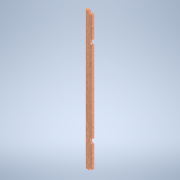
# Autodesk Inventor part: ReedRail
Saved by Autodesk Inventor 2022.2 (Build 262287000, 287)
## iProperties
Created: 2023-02-20
Part Number: ReedRail
Material: Wood (Oak)
Document SubType Name: Modeling
Designer: jaege
Density: 0.76 g/cm^3
Appearance: Red Oak - Natural Low Gloss
Author: jaege
Autodesk Inventor part; units mm, degrees
ref_plane "YZ Plane" through (0, 0, 0) normal (1, 0, 0) x (0, 1, 0)
ref_plane "XZ Plane" through (0, 0, 0) normal (0, 1, 0) x (-1, 0, 0)
ref_plane "XY Plane" through (0, 0, 0) normal (0, 0, 1) x (1, 0, 0)
sketch "Sketch1" plane through (0, 0, 0) normal (0, 0, 1) x (1, 0, 0)
  line L0 (0, 150.5) -> (7.5, 150.5) construction
  line L1 (15, 150.5) -> (15, -150.5)
  line L2 (15, -150.5) -> (7.5, -150.5)
  line L3 (0, -150.5) -> (0, 150.5)
  line L4 (0, 150.5) -> (7.5, 150.5) construction
  line L5 (7.5, 150.5) -> (7.5, 154.5)
  line L6 (7.5, 154.5) -> (0, 154.5)
  line L7 (0, 154.5) -> (0, 150.5)
  line L8 (0, -150.5) -> (7.5, -150.5) construction
  line L9 (7.5, -150.5) -> (7.5, -154.5)
  line L10 (7.5, -154.5) -> (0, -154.5)
  line L11 (0, -154.5) -> (0, -150.5)
  line L12 (7.5, -150.5) -> (0, -150.5) construction
  line L13 (7.5, 150.5) -> (15, 150.5)
  circle A0 centre (15, 96.116) radius 5.5796
  circle A1 centre (15, -96.116) radius 5.5796
  line L14 (-4.1159, 0) -> (24.6955, 0) construction
  point P0 (0, 0)
  point P1 (0, 0)
  point P2 (3.75, 150.5)
  point P3 (0, 0)
  point P4 (15, -101.6955)
  point P5 (15, -90.5364)
  point P6 (15, 90.5364)
  point P7 (15, 101.6955)
  dimension "d0" = 301
  dimension "d1" = 15
  dimension "d2" = 4
  dimension "d3" = 7.5
  dimension "d4" = 4
  dimension "d5" = 7.5
  dimension "d6" = 150.5
  constraints: 28 end point, 9 parallel, 4 horizontal, 4 perpendicular, 3 midpoint, 2 centre point, 2 point on line, 1 coincident, 1 equal radius, 1 symmetric about line
  measures "d0" distance of L3.start L0.start
  measures "d1" distance of L0.start L1.start
  measures "d2" distance of L0.end L5.end
  measures "d3" distance of L5.end L6.end
  measures "d4" distance of L2.end L9.end
  measures "d5" distance of L9.end L10.end
  measures "d6" vertical distance of point (3.75, 150.5) point (0, 0)
extrude "Extrusion1" add sketch "Sketch1" along normal blind 4 contours L1 A0 A1 L2 L9 L10 L11 L3 L7 L6 L5 L13
body "Solid1"
